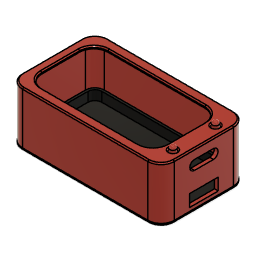
Lilygo+TDS3T+Case+B+v2_mod_dg v4 (Autodesk Fusion 360 design; units mm, degrees)
Autodesk Fusion 360 part; units mm, degrees
note: some values were not read from the file. Set by a fixed rule: which sketch regions a step uses.
sketch "Sketch1" plane through (0, 0, 0) normal (0, 1, 0) x (1, 0, 0) in component "Case"
  line L0 (-20.5, 14) -> (20.5, 14)
  line L1 (26.5, 8) -> (26.5, -8)
  line L2 (20.5, -14) -> (-20.5, -14)
  line L3 (-26.5, -8) -> (-26.5, 8)
  line L4 (-26.5, 14) -> (26.5, -14) construction
  line L5 (26.5, 14) -> (-26.5, -14) construction
  arc A0 (-20.5, 14) -> (-26.5, 8) centre (-20.5, 8) ccw
  arc A1 (-26.5, -8) -> (-20.5, -14) centre (-20.5, -8) ccw
  arc A2 (26.5, 8) -> (20.5, 14) centre (20.5, 8) ccw
  arc A3 (20.5, -14) -> (26.5, -8) centre (20.5, -8) ccw
  line L6 (-24.5, 16.5) -> (28.5, 16.5)
  line L7 (32.5, 12.5) -> (32.5, -12.5)
  line L8 (28.5, -16.5) -> (-24.5, -16.5)
  line L9 (-28.5, -12.5) -> (-28.5, 12.5)
  arc A4 (-24.5, 16.5) -> (-28.5, 12.5) centre (-24.5, 12.5) ccw
  arc A5 (32.5, 12.5) -> (28.5, 16.5) centre (28.5, 12.5) ccw
  arc A6 (28.5, -16.5) -> (32.5, -12.5) centre (28.5, -12.5) ccw
  arc A7 (-28.5, -12.5) -> (-24.5, -16.5) centre (-24.5, -12.5) ccw
  line L10 (-24.5, 18.1) -> (28.5, 18.1)
  arc A8 (34.1, 12.5) -> (28.5, 18.1) centre (28.5, 12.5) ccw
  line L11 (34.1, 12.5) -> (34.1, -12.5)
  arc A9 (28.5, -18.1) -> (34.1, -12.5) centre (28.5, -12.5) ccw
  line L12 (28.5, -18.1) -> (-24.5, -18.1)
  arc A10 (-30.1, -12.5) -> (-24.5, -18.1) centre (-24.5, -12.5) ccw
  line L13 (-30.1, -12.5) -> (-30.1, 12.5)
  arc A11 (-24.5, 18.1) -> (-30.1, 12.5) centre (-24.5, 12.5) ccw
  circle A12 centre (30, 9) radius 1.5
  circle A13 centre (30, -9) radius 1.5
  line L14 (26.5, 0) -> (32.5, 0) construction
  circle A14 centre (30, -9) radius 2.5
  circle A15 centre (30, 9) radius 2.5
  dimension "d1" = 53
  dimension "d3" = 6
  dimension "d4" = 6
  dimension "d18" = 6
  dimension "d19" = 2.5
  dimension "d20" = 2
  dimension "d21" = 2.5
  dimension "d22" = 28
  dimension "d23" = 4
  dimension "d24" = -1.6
  dimension "d31" = 3
  dimension "d32" = 3
  dimension "d82" = 1
  dimension "d83" = 1
  dimension "d84" = 9
  dimension "d85" = 9
  constraint horizontal L0
  constraint perpendicular L0 L1
  constraint parallel L0 L2
  constraint parallel L1 L3
  constraint coincident L4 origin
  constraint coincident L5 origin
  constraint coincident L4.start L0
  constraint coincident L4.start L3
  constraint tangent L0 A0
  constraint tangent L3 A0
  constraint coincident L5.end L2
  constraint coincident L5.end L3
  constraint tangent L2 A1
  constraint tangent L3 A1
  constraint equal A0 A1
  constraint coincident L5.start L0
  constraint coincident L5.start L1
  constraint tangent L0 A2
  constraint equal A0 A2
  constraint coincident L4.end L2
  constraint coincident L4.end L1
  constraint tangent L2 A3
  constraint horizontal L6
  constraint vertical L7
  constraint horizontal L8
  constraint vertical L9
  constraint tangent L6 A4
  constraint tangent L9 A4
  constraint tangent L6 A5
  constraint tangent L7 A5
  constraint equal A4 A5
  constraint tangent L8 A6
  constraint equal A4 A6
  constraint tangent L8 A7
  constraint tangent L9 A7
  constraint equal A4 A7
  constraint midpoint L1 L14.start
  constraint midpoint L7 L14.end
  constraint tangent L7 A6
  constraint tangent L1 A3
  constraint tangent L7 A14
  constraint tangent L7 A15
  constraint perpendicular L1 L14
  measures "d1" distance of L4.end L5.end
  measures "d3" radius of A0
  measures "d4" radius of A3
  measures "d18" distance of L1 L7
  measures "d19" distance of L0 L6
  measures "d20" distance of L3 L9
  measures "d21" distance of L2 L8
  measures "d22" distance of L0 L2
  measures "d23" radius of A4
  measures "d31" diameter of A12
  measures "d32" diameter of A13
  measures "d84" distance of A13.centre L14
  measures "d85" distance of A12.centre L14
extrude "Extrude1" add sketch "Sketch1" along normal blind 1 contours A14 | A15 | L6 L7 L8 L9 A4 A5 A6 A7 | L10 A8 L11 A9 L12 A10 L13 A11 makes body 1 in component "Case"
extrude "Extrude2" add sketch "Sketch1" against normal blind 21 contours L10 A8 L11 A9 L12 A10 L13 A11 bodies 1 in component "Case"
extrude "Extrude4" add sketch "Sketch1" against normal blind 3 contours A14 | A15 bodies 1 in component "Case"
chamfer "Chamfer1" distance 0.5 angle 45 1 faces at (8.1667, 1, 16.7333) on bodies 1 in component "Case"
sketch "Sketch2" plane through (34.1, 0, 0) normal (1, 0, 0) x (0, 0, -1) in component "Case"
  line L0 (12.5, 0.5) -> (-12.5, 0.5)
  line L1 (-12.5, 0.5) -> (-12.5, -21)
  line L2 (-12.5, -21) -> (12.5, -21)
  line L3 (12.5, -21) -> (12.5, 0.5)
  line L4 (-4, -7) -> (4, -7)
  arc A0 (4, -7) -> (4, -3) centre (4, -5) ccw
  line L5 (4, -3) -> (-4, -3)
  arc A1 (-4, -3) -> (-4, -7) centre (-4, -5) ccw
  line L6 (-4, -5) -> (4, -5) construction
  line L7 (0, 0) -> (0, -5) construction
  dimension "d95" = 8
  dimension "d96" = 2
  dimension "d28" = 5
  constraint tangent L4 A0
  constraint tangent A0 L5
  constraint parallel L4 L5
  constraint tangent L5 A1
  constraint tangent L4 A1
  constraint coincident A1.centre L6.start
  constraint coincident A0.centre L6.end
  constraint parallel L0 L6
  constraint coincident L7.start origin
  constraint midpoint L6 L7.end
  constraint vertical L7
  measures "d95" distance of A0.centre A1.centre
  measures "d96" radius of A1
  measures "d28" distance of L7.start L7.end
extrude "Extrude3" cut sketch "Sketch2" against normal blind 1.6 contours L4 A0 L5 A1 bodies 1 in component "Case"
sketch "Sketch1 (2)" plane through (0, 0, 0) normal (0, 1, 0) x (1, 0, 0) in component "Pushbutton"
  circle A0 centre (30, -9) radius 1.5 construction
  circle A1 centre (30, -9) radius 1.3
  line L0 (32.5, -12.5) -> (32.5, 12.5) construction
  line L1 (32.3, -12.5) -> (32.3, 12.5)
  line L2 (30, -11.5) -> (32.3, -11.5)
  line L3 (30, -6.5) -> (32.3, -6.5)
  arc A2 (30, -6.5) -> (30, -11.5) centre (30, -9) ccw
  dimension "d88" = -0.2
  dimension "d89" = -0.2
  dimension "d90" = 2.5
  constraint coincident L1 L2.end
  constraint perpendicular L1 L2
  constraint coincident L1 L3.end
  constraint perpendicular L1 L3
  constraint tangent L2 A2
  constraint coincident A0.centre A1.centre
  constraint tangent L3 A2
  measures "d90" radius of A2
extrude "Extrude1'" add sketch "Sketch1 (2)" against normal blind 1 separate body contours A1 | L1 L2 L3 A2 makes body 2 in component "Pushbutton"
extrude "Extrude2'" add sketch "Sketch1 (2)" along normal blind 6 contours A1 bodies 2 in component "Pushbutton"
chamfer "Chamfer1'" distance 0.5 angle 45 1 faces at (31.5333, -1, 9.8333) on bodies 2 in component "Pushbutton"
fillet "Fillet1" radius 1.3 1 edges at (28.788, 6, 9.4701) on bodies 2 in component "Pushbutton"
sketch "Sketch1 (3)" plane through (0, 0, 0) normal (0, 1, 0) x (1, 0, 0) in component "Base"
  line L0 (-22.5, 13) -> (15.5, 13)
  line L1 (15.5, 13) -> (15.5, 12)
  line L2 (15.5, 12) -> (-22.5, 12)
  line L3 (-22.5, 12) -> (-22.5, 13)
  line L4 (-22.5, -12) -> (5.5, -12)
  line L5 (5.5, -12) -> (5.5, -13)
  line L6 (5.5, -13) -> (-22.5, -13)
  line L7 (-22.5, -13) -> (-22.5, -12)
  arc A0 (-24.5, 16.5) -> (-28.5, 12.5) centre (-24.5, 12.5) ccw construction
  line L8 (-28.5, 12.5) -> (-28.5, -12.5) construction
  arc A1 (-28.5, -12.5) -> (-24.5, -16.5) centre (-24.5, -12.5) ccw construction
  line L9 (-24.5, -16.5) -> (28.5, -16.5) construction
  arc A2 (28.5, -16.5) -> (32.5, -12.5) centre (28.5, -12.5) ccw construction
  line L10 (32.5, -12.5) -> (32.5, 12.5) construction
  arc A3 (32.5, 12.5) -> (28.5, 16.5) centre (28.5, 12.5) ccw construction
  line L11 (28.5, 16.5) -> (-24.5, 16.5) construction
  arc A4 (34.1, 12.5) -> (28.5, 18.1) centre (28.5, 12.5) ccw
  line L12 (34.1, 12.5) -> (34.1, -12.5)
  arc A5 (28.5, -18.1) -> (34.1, -12.5) centre (28.5, -12.5) ccw
  line L13 (28.5, -18.1) -> (-24.5, -18.1)
  arc A6 (-30.1, -12.5) -> (-24.5, -18.1) centre (-24.5, -12.5) ccw
  line L14 (-30.1, -12.5) -> (-30.1, 12.5)
  arc A7 (-24.5, 18.1) -> (-30.1, 12.5) centre (-24.5, 12.5) ccw
  line L15 (-24.5, 18.1) -> (28.5, 18.1)
  line L16 (28.5, 16.4) -> (-24.5, 16.4)
  arc A8 (-24.5, 16.4) -> (-28.4, 12.5) centre (-24.5, 12.5) ccw
  line L17 (-28.4, 12.5) -> (-28.4, -12.5)
  arc A9 (-28.4, -12.5) -> (-24.5, -16.4) centre (-24.5, -12.5) ccw
  line L18 (-24.5, -16.4) -> (28.5, -16.4)
  arc A10 (28.5, -16.4) -> (32.4, -12.5) centre (28.5, -12.5) ccw
  arc A11 (32.4, 12.5) -> (28.5, 16.4) centre (28.5, 12.5) ccw
  line L19 (28.5, 15.4) -> (-24.5, 15.4)
  arc A12 (-24.5, 15.4) -> (-27.4, 12.5) centre (-24.5, 12.5) ccw
  line L20 (-27.4, 12.5) -> (-27.4, -12.5)
  arc A13 (-27.4, -12.5) -> (-24.5, -15.4) centre (-24.5, -12.5) ccw
  line L21 (-24.5, -15.4) -> (28.5, -15.4)
  arc A14 (28.5, -15.4) -> (31.4, -12.5) centre (28.5, -12.5) ccw
  line L22 (31.4, 11.5) -> (31.4, 12.5)
  arc A15 (31.4, 12.5) -> (28.5, 15.4) centre (28.5, 12.5) ccw
  line L23 (-28.4, 11.5) -> (-28.5, 11.5)
  line L24 (31.4, 12.5) -> (32.5, 12.5)
  line L25 (32.4, -12.5) -> (31.4, -12.5)
  dimension "d49_1" = 1
  dimension "d53_1" = 1
  dimension "d73" = 3.5
  dimension "d74" = 6
  dimension "d75" = 34
  dimension "d76" = 44
  dimension "d77" = 3.5
  constraint horizontal L0
  constraint vertical L1
  constraint horizontal L2
  constraint vertical L3
  constraint horizontal L4
  constraint vertical L5
  constraint horizontal L6
  constraint vertical L7
  constraint vertical L2.end L4.start
  constraint coincident L17 L23.start
  constraint coincident L8 L23.end
  constraint coincident L10.end A3.start
  constraint perpendicular L22 L25
  constraint concentric A0 A12
  constraint concentric A1 A13
  constraint concentric A2 A14
  constraint concentric A3 A15
  constraint tangent L22 A15
  constraint tangent A14 L22
  constraint tangent L21 A14
  constraint tangent A13 L21
  constraint tangent L19 A15
  constraint tangent L20 A13
  constraint tangent A12 L20
  constraint tangent L19 A12
  constraint concentric A0 A8
  constraint concentric A1 A9
  constraint concentric A2 A10
  constraint concentric A3 A11
  constraint tangent L18 A10
  constraint tangent L17 A9
  constraint tangent L16 A8
  constraint tangent A8 L17
  constraint tangent A9 L18
  constraint tangent L16 A11
  constraint horizontal A2.end A10.end
  measures "d49_1" distance of L0.start L2.end
  measures "d53_1" distance of L4.start L6.end
  measures "d73" distance of L6 L9
  measures "d74" distance of L6.end L8
  measures "d75" distance of L4.end L8
  measures "d76" distance of L1.end L8
  measures "d77" distance of L0 L11
extrude "Extrude1''" add sketch "Sketch1 (3)" against normal blind 1 separate body contours L0 L1 L2 L3 | L4 L5 L6 L7 | A4 L12 A5 L13 A6 L14 A7 L15 | L16 A8 L17 A9 L18 A10 A11 L19 A12 L20 A13 L21 A14 A15 L24 L25 makes body 3 in component "Base"
extrude "Extrude2''" add sketch "Sketch1 (3)" along normal blind 4 contours L16 A8 L17 A9 L18 A10 A11 L19 A12 L20 A13 L21 A14 A15 L24 L25 bodies 3 in component "Base"
extrude "Extrude3'" add sketch "Sketch1 (3)" against normal blind 1 bodies 3 in component "Base"
chamfer "Chamfer1''" distance 0.5 angle 45 1 faces at (10.8333, -1, -6.0333) on bodies 3 in component "Base"
ref_plane "WorkPlane2" through (-12.7, 2, 0) normal (1, 0, 0) x (0, 0, -1) in component "Base"
sketch "Sketch3" plane through (-12.7, 2, 0) normal (1, 0, 0) x (0, 0, -1) in component "Base"
  line L0 (0, -2) -> (0, 0) construction
  line L1 (-16.4, -0.0005) -> (-17.4, -0.0005)
  arc A0 (-16.4, 0.9995) -> (-17.4, -0.0005) centre (-16.4, -0.0005) ccw
  arc A1 (17.4, -0.0005) -> (16.4, 0.9995) centre (16.4, -0.0005) ccw
  line L2 (16.4, -0.0005) -> (17.4, -0.0005)
  line L3 (16.4, -2) -> (16.4, 2)
  line L4 (-16.4, -2) -> (-16.4, 2)
  line L5 (-16.4, -2) -> (16.4, -2) construction
  point P0 (-15.4, -2)
  point P1 (-15.4, 2)
  point P2 (15.4, -2)
  point P3 (15.4, 2)
  dimension "d101" = 2
  dimension "d103" = 2.0005
  constraint coincident L0.end origin
  constraint coincident L1.start A0.centre
  constraint symmetric L0 L1.start A1.centre
  constraint symmetric L0 L1.end A1.start
  constraint symmetric L0 A0.start A1.end
  constraint symmetric L0 A0 A1
  constraint coincident L4.start L5.start
  constraint coincident L3.start L5.end
  constraint coincident L0.start L5
  constraint perpendicular L0 L5
  constraint coincident L1.start L4
  constraint coincident A0.start L4
  constraint perpendicular L1 L4
  measures "d101" diameter of A0
  measures "d103" distance of L1.start L4.end
revolve "Revolve2" add sketch "Sketch3" angle 360 about axis through (-12.7, 1.9995, 16.4) along (0, 0, 1) separate body makes body 4 at (-12.7, 1.0081, 16.5305) makes body 5 at (-12.7, 1.0081, -16.5305) in component "Base"
copy_body "CopyPasteBodies1" bodies 4 5 makes body 6 makes body 7 in component "Base"
move_body "Move1" bodies 6 7 to x (1, 0, 0) y (0, 1, 0) z (0, 0, 1) at (29.4, 0, 0) in component "Base"
combine "Combine1" operation add target body 3 tool bodies 4 5 6 7 in component "Base"
combine "Combine3" operation cut target body 1 tool bodies 3 body 3 seen with x (1, 0, 0) y (0, 1, 0) z (0, 0, 1) at (0, -21, 0) keep tools in component "Case"
sketch "Skizze1" plane through (34.1, 0, 0) normal (1, 0, 0) x (0, 0, -1)
  line L0 (4, -7) -> (-4, -7)
  arc A0 (-4, -3) -> (-4, -7) centre (-4, -5) ccw
  line L1 (-4, -3) -> (4, -3)
  arc A1 (4, -7) -> (4, -3) centre (4, -5) ccw
  line L2 (12.5, 0.5) -> (-12.5, 0.5)
  line L3 (-12.5, 0.5) -> (-12.5, -21)
  line L4 (-12.5, -21) -> (12.5, -21)
  line L5 (12.5, -21) -> (12.5, 0.5)
  line L6 (12.5, -13) -> (-12.5, -13) construction
  line L7 (-12.5, -13) -> (-12.5, -21) construction
  line L8 (-12.5, -21) -> (12.5, -21) construction
  line L9 (12.5, -21) -> (12.5, -13) construction
  line L10 (-12.5, -13) -> (12.5, -21) construction
  line L11 (12.5, -13) -> (-12.5, -21) construction
  line L12 (6.05, -19.55) -> (-6.05, -19.55)
  line L13 (-6.05, -19.55) -> (-6.05, -14.45)
  line L14 (-6.05, -14.45) -> (6.05, -14.45)
  line L15 (6.05, -14.45) -> (6.05, -19.55)
  line L16 (6.05, -19.55) -> (-6.05, -14.45) construction
  line L17 (-6.05, -19.55) -> (6.05, -14.45) construction
  point P0 (0, -17)
  dimension "d106" = 6
  dimension "d107" = 12.1
  dimension "d108" = 5.1
  constraint horizontal L6
  constraint vertical L7
  constraint horizontal L8
  constraint vertical L9
  constraint coincident L3.end L4.start
  constraint coincident L5 L6.start
  constraint horizontal L12
  constraint perpendicular L12 L13
  constraint parallel L12 L14
  constraint parallel L13 L15
  constraint coincident L16 P0
  constraint coincident L17 P0
  constraint midpoint L11 P0
  measures "d106" distance of L0 L6
  measures "d107" distance of L13.end L14.end
  measures "d108" distance of L12.start L14.end
extrude "Extrusion5" cut sketch "Skizze1" against normal blind 7 contours L12 L13 L14 L15 bodies 1 in component "Case"
component "Case" placed x (1, 0, 0) y (0, 1, 0) z (0, 0, 1) at (0, 0, 0)
component "Pushbutton" placed x (1, 0, 0) y (0, 1, 0) z (0, 0, 1) at (0, -3, 0)
component "Pushbutton" placed x (1, 0, 0) y (0, 1, 0) z (0, 0, 1) at (0, -3, -18)
component "Base" placed x (1, 0, 0) y (0, 1, 0) z (0, 0, 1) at (0, -21, 0)
equation "d4 = d3"
equation "d19 = d21"
equation "d31 = d32"
equation "d73 = d77"
equation "d105 = 58.80 mm / 4"
